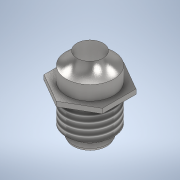
# Autodesk Inventor part: entrada_manguera
Saved by Autodesk Inventor 2022 (Build 260153000, 153)
## iProperties
Created: 2022-04-19
Part Number: entrada_manguera
Material: Generic
Document SubType Name: Modeling
Designer: ferna
Density: 1 g/cm^3
Appearance: Galvanized
Author: ferna
Autodesk Inventor part; units mm, degrees
ref_plane "YZ Plane" through (0, 0, 0) normal (1, 0, 0) x (0, 1, 0)
sketch "Sketch1" plane through (0, 0, 0) normal (0, 1, 0) x (-1, 0, 0)
  line L0 (12.25, -7.0725) -> (0, -14.1451)
  line L1 (0, -14.1451) -> (-12.25, -7.0725)
  line L2 (-12.25, -7.0725) -> (-12.25, 7.0725)
  line L3 (-12.25, 7.0725) -> (0, 14.1451)
  line L4 (0, 14.1451) -> (12.25, 7.0725)
  line L5 (12.25, 7.0725) -> (12.25, -7.0725)
  circle A0 centre (0, 0) radius 10
  dimension "d0" = 12.25
  dimension "d1" = 20
  constraints: 12 end point, 2 coincident, 1 centre point, 13 other
  measures "d0" distance from line of L5 point (0, 0)
  measures "d1" diameter of A0
extrude "Extrusion1" add sketch "Sketch1" along normal blind 2
sketch "Sketch2" plane through (0, 0, 0) normal (0, -1, 0) x (1, 0, 0)
  circle A0 centre (0, 0) radius 10
  constraints: 1 centre point, 1 coincident
extrude "Extrusion2" add sketch "Sketch2" against normal blind 8
sketch "Sketch3" plane through (0, 8, 0) normal (0, 1, 0) x (1, 0, 0)
  circle A0 centre (0, 0) radius 5
  dimension "d6" = 10
  constraints: 1 centre point, 1 coincident
  measures "d6" diameter of A0
extrude "Extrusion3" add sketch "Sketch3" along normal blind 8
fillet "Fillet1" radius 9.5 1 edges at (-5, 8, 0)
sketch "Sketch4" plane through (0, 0, 0) normal (0, -1, 0) x (1, 0, 0)
  circle A0 centre (0, 0) radius 10 projected
  circle A1 centre (0, 0) radius 10 projected
extrude "Extrusion4" add sketch "Sketch4" along normal blind 13
thread "Thread1" size "M20x2.5" class "6g" standard "ANSI Metric M Profile" full length
ref_plane "Work Plane1" through (0, -15, 0) normal (0, -1, 0) x (1, 0, 0)
sketch "Sketch5" plane through (0, -15, 0) normal (0, -1, 0) x (1, 0, 0)
  circle A0 centre (0, 0) radius 7.5
  dimension "d15" = 15
  constraints: 1 centre point, 1 coincident
  measures "d15" diameter of A0
loft "Loft1" add profiles "Sketch5" section 1 edges at (-10, -13, 0)
sketch "Sketch6" plane through (0, -15, 0) normal (0, -1, 0) x (1, 0, 0)
  circle A0 centre (0, 0) radius 7.5 projected
extrude "Extrusion5" add sketch "Sketch6" along normal blind 2
ref_plane "Work Plane2" through (0, -18, 0) normal (0, -1, 0) x (1, 0, 0)
sketch "Sketch7" plane through (0, -18, 0) normal (0, -1, 0) x (1, 0, 0)
  circle A0 centre (0, 0) radius 7
  dimension "d23" = 14
  constraints: 1 centre point, 1 coincident
  measures "d23" diameter of A0
loft "Loft2" add profiles "Sketch7" section 1 edges at (-7.5, -17, 0)
sketch "Sketch8" plane through (0, -18, 0) normal (0, -1, 0) x (1, 0, 0)
  circle A0 centre (0, 0) radius 5.5
  dimension "d28" = 11
  constraints: 1 centre point, 1 coincident
  measures "d28" diameter of A0
extrude "Extrusion6" cut sketch "Sketch8" against normal through all
sketch "Sketch9" plane through (0, -18, 0) normal (0, -1, 0) x (1, 0, 0)
  circle A0 centre (0, 0) radius 5.5 projected
body "Solid1"
